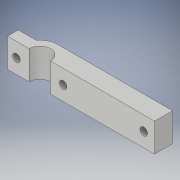
# Autodesk Inventor part: outerCrutchAttacement
Saved by Autodesk Inventor 2017 SP1 (Build 210196100, 196)
## iProperties
Created: 2016-07-31
Part Number: outerCrutchAttacement
Material: Generic
Document SubType Name: Modeling
Designer: steele
Density: 1 g/cm^3
Appearance: Default
Author: steele
Autodesk Inventor part; units mm, degrees
ref_plane "YZ Plane" through (0, 0, 0) normal (1, 0, 0) x (0, 1, 0)
ref_plane "XZ Plane" through (0, 0, 0) normal (0, 1, 0) x (-1, 0, 0)
ref_plane "XY Plane" through (0, 0, 0) normal (0, 0, 1) x (1, 0, 0)
sketch "Sketch1" plane through (0, 0, 0) normal (0, 1, 0) x (-1, 0, 0)
  line L0 (0, 0) -> (0, 38.1) construction
  line L1 (0, 0) -> (0, -38.1) construction
  arc A0 (-9.525, -38.1) -> (9.525, -38.1) centre (0, -38.1) ccw construction
  circle A1 centre (0, 38.1) radius 9.525 construction
  arc A2 (-9.525, -38.1) -> (9.525, -38.1) centre (0, -38.1) ccw
  arc A3 (0, -53.975) -> (12.7, -47.625) centre (0, -38.1) ccw
  line L2 (15.875, -38.1) -> (28.575, -38.1)
  line L3 (28.575, -38.1) -> (28.575, -47.625)
  line L4 (28.575, -47.625) -> (12.7, -47.625)
  line L5 (-15.875, -38.1) -> (-101.6, -38.1)
  line L6 (-101.6, -38.1) -> (-101.6, -53.975)
  line L7 (-101.6, -53.975) -> (0, -53.975)
  line L8 (15.875, -38.1) -> (-15.875, -38.1) construction
  line L9 (15.875, -38.1) -> (9.525, -38.1)
  line L10 (-9.525, -38.1) -> (-15.875, -38.1)
  dimension "d0" = 76.2
  dimension "d1" = 19.05
  dimension "d2" = 31.75
  dimension "d3" = 12.7
  dimension "d4" = 9.525
  dimension "d5" = 101.6
  constraints: 22 end point, 6 point on circle, 4 centre point, 4 coincident, 3 collinear, 3 horizontal, 3 perpendicular, 2 equal radius, 2 point on line, 2 vertical, 1 parallel, 1 tangent
  measures "d0" distance of L0.end L1.end
  measures "d1" diameter of A0
  measures "d2" diameter of A3
  measures "d3" distance of L2.start L2.end
  measures "d4" distance of L2.end L3.end
  measures "d5" distance of L7.end L6.end
extrude "Extrusion1" add sketch "Sketch1" along normal mid plane 25.4
sketch "Sketch2" plane through (-12.7, 12.7, -47.625) normal (0, 0, -1) x (-1, 0, 0)
  line L0 (15.875, 0) -> (15.875, -25.4) construction
  line L1 (0, 0) -> (-12.7, 0) construction
  line L2 (15.875, -25.4) -> (0, 0) construction
  line L3 (0, 0) -> (0, -25.4) construction
  line L4 (0, -25.4) -> (15.875, 0) construction
  point P0 (-12.7, -12.7)
  point P1 (7.9375, -12.7)
  constraints: 4 end point, 1 midpoint
hole "Hole1" at (-20.6375, 0, -47.625) direction (0, 0, 1) diameter 6.7564 end through all clearance for "Flat Head Machine Screw (82)" size "1/4" standard "Ansi Unified Screw Threads"
sketch "Sketch3" plane through (101.6, 12.7, -53.975) normal (0, 0, -1) x (-1, 0, 0)
  line L0 (0, 0) -> (0, -25.4) construction
  line L1 (0, -12.7) -> (101.6, -12.7) construction
  line L2 (92.075, 0) -> (0, 0) construction
  line L3 (9.525, 0) -> (9.525, -25.4) construction
  point P0 (9.525, -12.7)
  dimension "d15" = 9.525
  constraints: 4 end point, 2 midpoint, 1 horizontal, 1 point on line, 1 vertical
  measures "d15" distance between parallel lines of L3 L0
hole "Hole2" at (92.075, 0, -53.975) direction (0, 0, 1) diameter 6.7564 end through all clearance for "Flat Head Machine Screw (82)" size "1/4" standard "Ansi Unified Screw Threads"
sketch "Sketch4" plane through (101.6, 12.7, -53.975) normal (0, 0, -1) x (-1, 0, 0)
  point P0 (80.9625, -12.7)
hole "Hole3" at (20.6375, 0, -53.975) direction (0, 0, 1) diameter 6.7564 depth 15.875
equation "\"d0\" = crutchTubSpacing"
equation "\"d1\" = cruchTubeDiam"
equation "\"d2\" = cruchTubeDiam + 2 * wallThickness"
equation "\"cruchTubeDiam\" = 19.05"
equation "\"wallThickness\" = 6.35"
equation "\"crutchTubSpacing\" = 76.2"
equation "\"supportHeight\" = 25.4"
body "Solid1"
